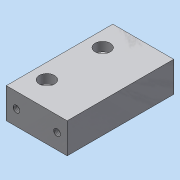
# Autodesk Inventor part: BC-10012
Saved by Autodesk Inventor 2016 (Build 200138000, 138)
## iProperties
Created: 2015-11-26
Part Number: BC-10012
Project: DIPOLO BC-3T- SIRIUS
Cost Center: 1504002005
Material: Alumínio 7075
Document SubType Name: Modeling
Designer: reinaldo.basilio
Mass: 507.363 g
Surface Area: 258.079 cm^2
Volume: 180.556 cm^3
Density: 2.81 g/cm^3
Appearance: Satin - Brushed Heavy
Description: Espaçador
RuleStatus: InUse
AfterMaterialChange0: file://_iMaterial
AfterAnyiPropertyChange0: file://_iMaterial
AfterDocNew0: file://_Naming_par
AfterDocNew1: file://_NameStart
AfterDocNew2: file://_NameStart1
AfterDocNew3: file://_Materiais
DocNumber: XXXXX-XXX-XXXX-00-001.ipt
Folder: .
Title: DIPOLO BC-3T- SIRIUS
Author: reinaldo.basilio
Subject: BC-10012
Autodesk Inventor part; units mm, degrees
ref_plane "YZ Plane" through (0, 0, 0) normal (1, 0, 0) x (0, 1, 0)
ref_plane "XZ Plane" through (0, 0, 0) normal (0, 1, 0) x (-1, 0, 0)
ref_plane "XY Plane" through (0, 0, 0) normal (0, 0, 1) x (1, 0, 0)
sketch "Sketch5" plane through (0, 0, 0) normal (0, 0, 1) x (1, 0, 0)
  line L0 (-52.5, 30) -> (52.5, 30)
  line L1 (52.5, 30) -> (52.5, -30)
  line L2 (52.5, -30) -> (-52.5, -30)
  line L3 (-52.5, -30) -> (-52.5, 30)
  point P0 (0, 0)
  point P1 (0, 30)
  point P2 (52.5, 0)
  dimension "d8" = 60
  dimension "d9" = 105
  constraints: 8 end point, 2 midpoint, 2 parallel, 1 horizontal, 1 horizontal alignment, 1 perpendicular, 1 vertical alignment
  measures "d8" distance of L2.end L0.start
  measures "d9" distance of L0.start L0.end
extrude "Extrusion5" add sketch "Sketch5" along normal blind 30
sketch "Sketch6" plane through (0, 0, 30) normal (0, 0, 1) x (1, 0, 0)
  circle A0 centre (-27.5, -15) radius 4
  circle A1 centre (27.5, -15) radius 4
  line L0 (-52.5, -30) -> (52.5, -30) projected
  point P0 (0, 0)
  dimension "d12" = 55
  dimension "d13" = 27.5
  dimension "d14" = 8
  dimension "d39" = 15
  constraints: 2 centre point, 1 equal radius, 1 horizontal alignment
  measures "d12" distance of A1.centre A0.centre
  measures "d13" horizontal distance of point (0, 0) A0.centre
  measures "d14" diameter of A0
  measures "d39" distance from line of A1.centre L0
hole "Hole1" at (-27.5, -15, 30) at (27.5, -15, 30) direction (0, 0, -1) diameter 9 end through all counterbore diameter 15 counterbore depth 9 clearance for "Socket Head Cap Screw DIN EN ISO 4762" size "M8" standard "DIN"
sketch "Sketch7" plane through (-52.5, -30, 0) normal (-1, 0, 0) x (0, 0, 1)
  line L0 (0, 0) -> (30, 0) projected
  line L1 (0, 60) -> (30, 60) projected
  circle A0 centre (15, 50) radius 4
  circle A1 centre (15, 10) radius 4
  point P0 (0, 30)
  point P1 (15, 60)
  point P2 (15, 0)
  dimension "d22" = 40
  dimension "d23" = 20
  dimension "d24" = 8
  constraints: 2 centre point, 2 midpoint, 2 vertical alignment, 1 equal radius
  measures "d22" distance of A1.centre A0.centre
  measures "d23" vertical distance of point (0, 30) A0.centre
  measures "d24" diameter of A0
hole "Hole2" at (-52.5, 20, 15) at (-52.5, -20, 15) direction (1, 0, 0) diameter 6.647 depth 18 tip angle 118 thread size "M8x1.25" class "6H" standard "ISO Metric profile"
sketch "Sketch8" plane through (52.5, -30, 0) normal (1, 0, 0) x (0, 0, -1)
  circle A0 centre (-15, 10) radius 3.3235
  circle A1 centre (-15, 50) radius 3.3235
  circle A2 centre (-15, 10) radius 3.3235 projected
  circle A3 centre (-15, 50) radius 3.3235 projected
  point P0 (0, 30)
  constraints: 4 concentric, 2 centre point
hole "Hole3" at (52.5, -20, 15) at (52.5, 20, 15) direction (-1, 0, 0) diameter 6.647 depth 18 tip angle 118 thread size "M8x1.25" class "6H" standard "ISO Metric profile"
equation "\"d13\" = 0.5 * d12"
equation "\"d23\" = 0.5 * d22"
body "Solid5"
